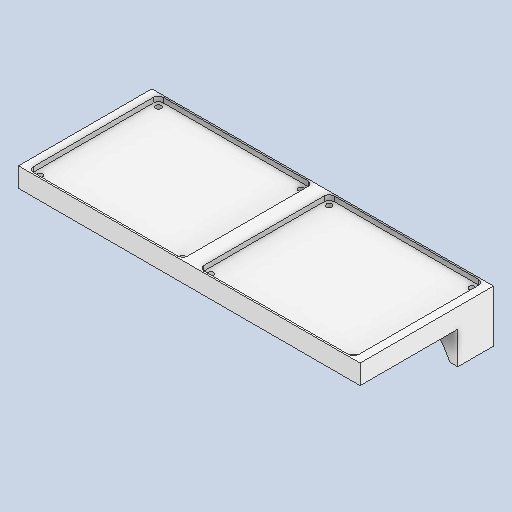
# Autodesk Inventor part: motor_driver_frame
Saved by Autodesk Inventor 2025.3 (Build 293356030, 356C)
## iProperties
Created: 2025-09-19
Part Number: motor_driver_frame
Material: PLA+ filament
Document SubType Name: Modeling
Designer: MSI
Density: 1.23 g/cm^3
Appearance: 일반
Mass: 217.118 g
Surface Area: 497.076 cm^2
Volume: 176.519 cm^3
Author: MSI
Autodesk Inventor part; units mm, degrees
ref_plane "YZ Plane" through (0, 0, 0) normal (1, 0, 0) x (0, 1, 0)
ref_plane "XZ Plane" through (0, 0, 0) normal (0, 1, 0) x (-1, 0, 0)
ref_plane "XY Plane" through (0, 0, 0) normal (0, 0, 1) x (1, 0, 0)
sketch "스케치1" plane through (0, 0, 0) normal (0, 0, 1) x (1, 0, 0)
  line L0 (-105, 16) -> (105, 16)
  line L1 (105, 16) -> (105, -16)
  line L2 (105, -16) -> (-105, -16)
  line L3 (-105, -16) -> (-105, 16)
  line L4 (-105, 16) -> (105, -16) construction
  line L5 (105, 16) -> (-105, -16) construction
  point P0 (0, 0)
  dimension "d0" = 210
  dimension "d1" = 32
  constraints: 12 end point, 2 midpoint, 2 parallel, 1 horizontal, 1 perpendicular
  measures "d0" distance of L1.end L2.end
  measures "d1" distance of L0.end L1.end
extrude "돌출1" add sketch "스케치1" along normal mid plane 82
sketch "스케치2" plane through (0, 0, 41) normal (0, 0, 1) x (1, 0, 0)
  circle A0 centre (-60, -36) radius 45
  line L0 (105, 16) -> (-105, 16) projected
  line L1 (0, 16) -> (0, -16)
  line L2 (-105, -16) -> (105, -16) projected
  circle A1 centre (60, -36) radius 45
  point P0 (0, 0)
  dimension "d4" = 90
  dimension "d5" = 60
  dimension "d6" = 52
  constraints: 2 centre point, 2 end point, 2 midpoint, 1 symmetric about line, 1 other
  measures "d4" diameter of A0
  measures "d5" horizontal distance of point (0, 0) A0.centre
  measures "d6" distance from line of L0 A0.centre
extrude "돌출2" cut sketch "스케치2" against normal through all
sketch "스케치3" plane through (0, 0, 41) normal (0, 0, 1) x (1, 0, 0)
  line L0 (-105, -16) -> (-105, 16) projected
  line L1 (-105, 4) -> (105, 4)
  line L2 (105, 4) -> (105, -16)
  line L3 (105, -16) -> (-105, -16)
  line L4 (-105, -16) -> (-105, 4)
  arc A0 (-19.6887, -16) -> (-100.3113, -16) centre (-60, -36) ccw projected
  line L5 (-19.6887, -16) -> (19.6887, -16) projected
  point P0 (0, 0)
  point P1 (0, 4)
  dimension "d11" = 20
  constraints: 8 end point, 2 parallel, 1 collinear, 1 horizontal, 1 midpoint, 1 perpendicular, 1 point on line, 1 vertical alignment
  measures "d11" distance between parallel lines of L3 L1
extrude "돌출3" cut sketch "스케치3" against normal blind 60 contours L0 L1 A0 L3 | A0 L1 L3 | A0 L1 L2 L3
sketch "스케치7" plane through (0, 0, 41) normal (0, 0, 1) x (1, 0, 0)
  line L0 (-105, -16) -> (-105, 16) projected
  line L1 (80.6155, 4) -> (105, 4) projected
  line L2 (-105, 16) -> (105, 16)
  line L3 (105, 16) -> (105, 4)
  line L4 (105, 4) -> (-105, 4)
  line L5 (-105, 4) -> (-105, 16)
  point P0 (0, 0)
  constraints: 8 end point, 2 parallel, 1 horizontal, 1 perpendicular
extrude "돌출5" add sketch "스케치7" against normal blind 15
sketch "스케치4" plane through (-105, 16, 41) normal (0, 1, 0) x (1, 0, 0)
  line L0 (0, 82) -> (210, 82) projected
  line L1 (65.6155, 0) -> (144.3845, 0) projected
  line L2 (5, 81) -> (100, 81)
  line L3 (100, 81) -> (100, 1)
  line L4 (100, 1) -> (5, 1)
  line L5 (5, 1) -> (5, 81)
  line L6 (0, 82) -> (0, 0) projected
  line L7 (0, 82) -> (105, 82) construction
  point P0 (52.5, 82)
  point P1 (52.5, 81)
  point P2 (0, 41)
  point P3 (5, 41)
  dimension "d12" = 80
  dimension "d13" = 95
  constraints: 10 end point, 5 midpoint, 2 parallel, 1 collinear, 1 horizontal, 1 horizontal alignment, 1 perpendicular, 1 vertical alignment
  measures "d12" distance of L4.end L2.start
  measures "d13" distance of L3.end L4.end
extrude "돌출4" cut sketch "스케치4" against normal blind 3
fillet "모깎기1" radius 3 4 edges at (-5, 14.5, -40) (-5, 14.5, 40) (-100, 14.5, -40) (-100, 14.5, 40)
sketch "스케치5" plane through (-105, 13, 41) normal (0, 1, 0) x (1, 0, 0)
  arc A0 (5, 4) -> (8, 1) centre (8, 4) ccw construction
  line L0 (97, 1) -> (8, 1) construction
  arc A1 (97, 1) -> (100, 4) centre (97, 4) ccw construction
  line L1 (100, 78) -> (100, 4) construction
  arc A2 (100, 78) -> (97, 81) centre (97, 78) ccw construction
  line L2 (8, 81) -> (97, 81) construction
  arc A3 (8, 81) -> (5, 78) centre (8, 78) ccw construction
  line L3 (5, 4) -> (5, 78) construction
  line L4 (8.66, 77.37) -> (96.34, 77.37) construction
  line L5 (96.34, 77.37) -> (96.34, 4.63) construction
  line L6 (96.34, 4.63) -> (8.66, 4.63) construction
  line L7 (8.66, 4.63) -> (8.66, 77.37) construction
  line L8 (8.66, 77.37) -> (96.34, 4.63) construction
  line L9 (96.34, 77.37) -> (8.66, 4.63) construction
  line L10 (5, 4) -> (5, 78) construction
  line L11 (8, 81) -> (97, 81) construction
  point P0 (105, 41)
  point P1 (52.5, 41)
  point P2 (5, 41)
  point P3 (52.5, 81)
  dimension "d18" = 87.68
  dimension "d19" = 72.74
  constraints: 12 end point, 4 midpoint, 2 parallel, 1 horizontal, 1 horizontal alignment, 1 perpendicular, 1 vertical alignment
  measures "d18" distance of L5.end L6.end
  measures "d19" distance of L6.end L4.start
hole "구멍1" at (-96.34, 13, -36.37) at (-96.34, 13, 36.37) at (-8.66, 13, -36.37) at (-8.66, 13, 36.37) direction (0, -1, 0) diameter 3.4 depth 8 tip angle 118 clearance for "Flat Head Machine Screw" size "M3" standard "Ansi Metric M Profile"
mirror "미러1" about plane through (0, 0, 0) normal (1, 0, 0) of "돌출4", "모깎기1", "구멍1"
sketch "스케치6" plane through (0, 0, -19) normal (0, 0, 1) x (1, 0, 0)
  line L0 (-12.5, -11) -> (12.5, -11) construction
  line L1 (19.6887, -16) -> (-19.6887, -16) projected
  point P0 (0, 0)
  point P1 (0, -11)
  dimension "d27" = 5
  dimension "d28" = 25
  constraints: 2 end point, 1 horizontal, 1 midpoint, 1 vertical alignment
  measures "d27" distance between parallel lines of L0 L1
  measures "d28" distance of L0.start L0.end
hole "구멍2" at (-12.5, -11, -19) at (12.5, -11, -19) direction (0, 0, -1) diameter 3.4 end through all clearance for "Flat Head Machine Screw" size "M3" standard "Ansi Metric M Profile"
